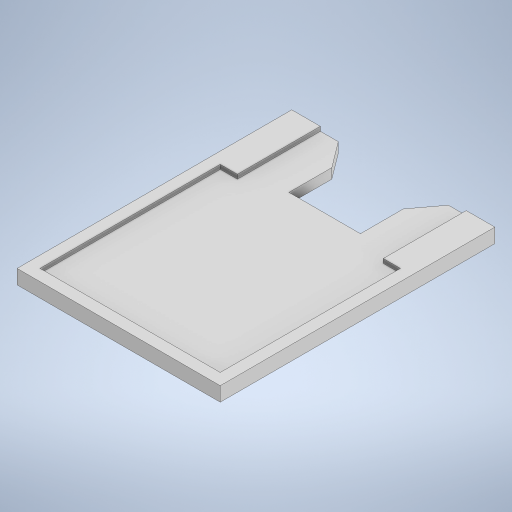
# Autodesk Inventor part: Bauteil2
Saved by Autodesk Inventor 2023.1 (Build 271208000, 208)
## iProperties
Created: 2023-04-26
Part Number: Bauteil2
Material: Generisch
Document SubType Name: Sheet Metal
Designer: marco
Density: 1 g/cm^3
Sheet Metal Rule: Standard_mm
Appearance: Vorgabe
Author: marco
Autodesk Inventor part; units mm, degrees
ref_plane "YZ Plane" through (0, 0, 0) normal (1, 0, 0) x (0, 1, 0)
ref_plane "XZ Plane" through (0, 0, 0) normal (0, 1, 0) x (-1, 0, 0)
ref_plane "XY Plane" through (0, 0, 0) normal (0, 0, 1) x (1, 0, 0)
sketch "Skizze1" plane through (0, 0, 0) normal (0, 1, 0) x (-1, 0, 0)
  line L0 (0, 0) -> (63, 0)
  line L1 (63, 0) -> (63, -63)
  line L2 (63, -63) -> (0, -63)
  line L3 (0, -63) -> (0, 0)
  line L4 (-4, 4) -> (67, 4)
  line L5 (67, 4) -> (67, -92)
  line L6 (67, -92) -> (-4, -92)
  line L7 (-4, -92) -> (-4, 4)
  line L8 (57, -63) -> (6, -63)
  line L9 (6, -63) -> (6, -68)
  line L10 (6, -68) -> (57, -68)
  line L11 (57, -68) -> (57, -63)
  line L12 (44, -68) -> (19, -68)
  line L13 (19, -68) -> (19, -92)
  line L14 (19, -92) -> (44, -92)
  line L15 (44, -92) -> (44, -68)
  line L16 (44, -68) -> (44, -83)
  line L17 (44, -83) -> (44, -93)
  line L18 (44, -93) -> (49.7342, -93)
  line L19 (49.7342, -93) -> (44, -83)
  line L20 (49.1608, -92) -> (44, -92)
  line L21 (19, -83) -> (19, -93)
  line L22 (19, -93) -> (11.5, -93)
  line L23 (11.5, -93) -> (19, -83)
  line L24 (12.25, -92) -> (19, -92)
  line L25 (57, -68) -> (57, -71.1865)
  line L26 (57, -71.1865) -> (57, -92)
  line L27 (6, -68) -> (6, -92)
  point P0 (19, -80)
  dimension "d0" = 63
  dimension "d1" = 63
  dimension "d2" = 71
  dimension "d3" = 96
  dimension "d4" = 51
  dimension "d5" = 5
  dimension "d6" = 6
  dimension "d7" = 6
  dimension "d8" = 4
  dimension "d9" = 25
  dimension "d10" = 24
  dimension "d11" = 15
  dimension "d14" = 10
  dimension "d15" = 10
  dimension "d16" = 15
  dimension "d23" = 13
  dimension "d24" = 13
  constraints: 56 end point, 14 point on line, 10 parallel, 6 perpendicular, 4 horizontal, 1 collinear, 1 midpoint
  measures "d0" distance of L1.end L2.end
  measures "d1" distance of L0.end L1.end
  measures "d2" distance of L5.end L6.end
  measures "d3" distance of L4.end L5.end
  measures "d4" distance of L10.end L9.end
  measures "d5" distance of L9.end L8.end
  measures "d6" distance between parallel lines of L1 L11
  measures "d7" distance between parallel lines of L9 L3
  measures "d8" distance between parallel lines of L4 L0
  measures "d9" distance of L14.end L13.end
  measures "d10" distance of L12.end L13.end
  measures "d11" distance of L12.start L16.end
  measures "d14" distance of L16.end L17.end
  measures "d15" distance of L21.start L21.end
  measures "d16" distance from line of L10 L21.start
  measures "d23" distance from line of L27 point (19, -80)
  measures "d24" distance between parallel lines of L26 L15
extrude "Extrusion1" add sketch "Skizze1" along normal blind 1.5 contours L3 L2 L9 L27 L6 L7 L4 L5 L26 L25 L11 L1 L0
sketch "Skizze2" plane through (0, 0, 0) normal (0, -1, 0) x (1, 0, 0)
  line L0 (4, 4) -> (4, -92) projected
  line L1 (-57, -92) -> (-67, -92) projected
  line L2 (4, 4) -> (-67, 4)
  line L3 (-67, 4) -> (-67, -92)
  line L4 (-67, -92) -> (4, -92)
  line L5 (4, -92) -> (4, 4)
  line L6 (-19, -92) -> (-44, -92)
  line L7 (-44, -92) -> (-44, -68)
  line L8 (-44, -68) -> (-19, -68)
  line L9 (-19, -68) -> (-19, -92)
  line L10 (-6, -92) -> (-6, -63) projected
  line L11 (-57, -63) -> (-57, -92) projected
  line L12 (-44, -68) -> (-44, -83)
  line L13 (-44, -83) -> (-44, -92)
  line L14 (-44, -83) -> (-44, -93)
  line L15 (-44, -83) -> (-34, -83) construction
  line L16 (-44, -93) -> (-51.5, -93)
  line L17 (-51.5, -93) -> (-44, -83)
  line L18 (-19, -83) -> (-19, -93)
  line L19 (-19, -93) -> (-11.5, -93)
  line L20 (-11.5, -93) -> (-19, -83)
  point P0 (0, 0)
  point P1 (-50.75, -92)
  point P2 (-12.25, -92)
  dimension "d19" = 25
  dimension "d20" = 24
  dimension "d21" = 13
  dimension "d22" = 13
  dimension "d25" = 15
  dimension "d26" = 10
  dimension "d27" = 90
  dimension "d28" = 7.5
  dimension "d29" = 7.5
  constraints: 34 end point, 6 point on line, 5 parallel, 3 horizontal, 3 perpendicular, 2 collinear
  measures "d19" distance of L7.end L8.end
  measures "d20" distance of L6.end L7.end
  measures "d21" distance between parallel lines of L10 L9
  measures "d22" distance between parallel lines of L11 L7
  measures "d25" distance of L7.end L12.end
  measures "d26" distance of L12.end L14.end
  measures "d27" angle of L14 L15
  measures "d28" distance of L14.end L16.end
  measures "d29" distance of L18.end L19.end
extrude "Extrusion2" add sketch "Skizze2" along normal blind 3.5 contours L0 L4 L20 L9 L8 L7 L17 L1 L3 L2
equation "\"d15\" = d14"
equation "\"Biegeradius\" = Stärke"
equation "\"BreiteBiegungsfreistellung\" = Stärke"
equation "\"TiefeBiegungsfreistellung\" = 0.5 * Stärke"
equation "\"GrößeEckenfreistellung\" = 4 * Stärke"
equation "\"MinimalRest\" = 2 * Stärke"
equation "\"Übergangsradius\" = Biegeradius"
equation "\"JacobiRadiusGröße\" = Biegeradius"
equation "\"Abstandsgröße\" = Stärke"
equation "\"Stärke\" = 0.5"
